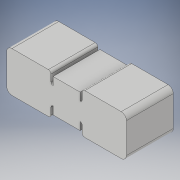
# Autodesk Inventor part: ARTHURw5.5bAutomobloxConnectorPiece
Saved by Autodesk Inventor 2018 (Build 220112000, 112)
## iProperties
Created: 2019-01-22
Part Number: ARTHURw5.5bAutomobloxConnectorPiece
Material: Generic
Document SubType Name: Modeling
Designer: russd
Density: 1 g/cm^3
Appearance: Default
Author: russd
Autodesk Inventor part; units mm, degrees
ref_plane "YZ Plane" through (0, 0, 0) normal (1, 0, 0) x (0, 1, 0)
ref_plane "XZ Plane" through (0, 0, 0) normal (0, 1, 0) x (-1, 0, 0)
ref_plane "XY Plane" through (0, 0, 0) normal (0, 0, 1) x (1, 0, 0)
sketch "Sketch1" plane through (0, 0, 0) normal (0, 0, 1) x (1, 0, 0)
  line L0 (-26.67, 9.906) -> (-8.89, 9.906)
  line L1 (-7.62, 8.636) -> (-7.62, 5.334)
  line L2 (-6.604, 4.318) -> (-6.604, 4.318)
  line L3 (-6.604, 4.318) -> (-6.604, 8.128)
  line L4 (-6.604, 8.128) -> (0, 8.128)
  line L5 (-29.21, 7.366) -> (-29.21, 0)
  line L6 (0, 8.128) -> (0, 0)
  line L7 (0, 0) -> (-29.21, 0)
  arc A0 (-7.62, 5.334) -> (-6.604, 4.318) centre (-6.604, 5.334) ccw
  arc A1 (-7.62, 8.636) -> (-8.89, 9.906) centre (-8.89, 8.636) ccw
  arc A2 (-26.67, 9.906) -> (-29.21, 7.366) centre (-26.67, 7.366) ccw
  line L8 (26.67, 9.906) -> (8.89, 9.906)
  line L9 (7.62, 8.636) -> (7.62, 5.334)
  line L10 (6.604, 4.318) -> (6.604, 4.318)
  line L11 (6.604, 4.318) -> (6.604, 8.128)
  line L12 (6.604, 8.128) -> (0, 8.128)
  line L13 (29.21, 7.366) -> (29.21, 0)
  line L14 (0, 0) -> (29.21, 0)
  arc A3 (6.604, 4.318) -> (7.62, 5.334) centre (6.604, 5.334) ccw
  arc A4 (8.89, 9.906) -> (7.62, 8.636) centre (8.89, 8.636) ccw
  arc A5 (29.21, 7.366) -> (26.67, 9.906) centre (26.67, 7.366) ccw
  line L15 (-26.67, -9.906) -> (-8.89, -9.906)
  line L16 (-7.62, -8.636) -> (-7.62, -8.128)
  line L17 (-6.604, -4.318) -> (-6.604, -8.128)
  line L18 (-6.604, -8.128) -> (0, -8.128)
  line L19 (-29.21, -7.366) -> (-29.21, 0)
  line L20 (0, -8.128) -> (0, 0)
  arc A6 (-8.89, -9.906) -> (-7.62, -8.636) centre (-8.89, -8.636) ccw
  arc A7 (-29.21, -7.366) -> (-26.67, -9.906) centre (-26.67, -7.366) ccw
  line L21 (29.21, -7.366) -> (29.21, 0)
  arc A8 (26.67, -9.906) -> (29.21, -7.366) centre (26.67, -7.366) ccw
  line L22 (26.67, -9.906) -> (8.89, -9.906)
  arc A9 (7.62, -8.636) -> (8.89, -9.906) centre (8.89, -8.636) ccw
  line L23 (6.604, -4.318) -> (6.604, -8.128)
  line L24 (6.604, -8.128) -> (0, -8.128)
  line L25 (-7.62, -8.636) -> (-7.62, -5.334)
  line L26 (-7.62, -5.334) -> (-7.62, -5.334)
  line L27 (-6.604, -4.318) -> (-6.604, -4.318)
  arc A10 (-6.604, -4.318) -> (-7.62, -5.334) centre (-6.604, -5.334) ccw
  line L28 (7.62, -8.636) -> (7.62, -5.334)
  line L29 (7.62, -5.334) -> (7.62, -5.334)
  line L30 (6.604, -4.318) -> (6.604, -4.318)
  arc A11 (7.62, -5.334) -> (6.604, -4.318) centre (6.604, -5.334) ccw
  point P0 (-7.62, -4.318)
  dimension "d0" = 29.21
  dimension "d1" = 7.62
  dimension "d2" = 1.016
  dimension "d3" = 5.588
  dimension "d4" = 9.906
  dimension "d5" = 8.128
  dimension "d6" = 1.016
  dimension "d7" = 1.27
  dimension "d8" = 2.54
  dimension "d9" = 1.016
  dimension "d10" = 1.016
  constraints: 62 end point, 31 symmetric about line, 24 point on circle, 12 centre point, 10 tangent, 7 perpendicular, 5 vertical, 4 point on line, 1 horizontal, 7 other
  measures "d0" distance between parallel lines of L6 L5
  measures "d1" distance from line of L4.end L1
  measures "d2" distance between parallel lines of L3 L1
  measures "d3" distance between parallel lines of L0 L2
  measures "d4" distance between parallel lines of L7 L0
  measures "d5" distance between parallel lines of L7 L4
  measures "d6" radius of A0
  measures "d7" radius of A1
  measures "d8" radius of A2
  measures "d9" radius of A10
  measures "d10" radius of A11
extrude "Extrusion1" add sketch "Sketch1" along normal blind 22.86
body "Solid1"
